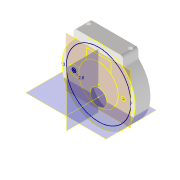
# Autodesk Inventor part: Pump_Base_Motor_tubeholder_new
Saved by Autodesk Inventor 2022.5 (Build 265521000, 521)
## iProperties
Created: 2023-11-14
Part Number: Pump_Base_Motor_tubeholder_new
Material: Generisch
Document SubType Name: Modeling
Designer: diederichbenedict
Density: 1 g/cm^3
Appearance: Vorgabe
Author: diederichbenedict
Autodesk Inventor part; units mm, degrees
ref_plane "YZ Plane" through (0, 0, 0) normal (1, 0, 0) x (0, 1, 0)
ref_plane "XZ Plane" through (0, 0, 0) normal (0, 1, 0) x (-1, 0, 0)
ref_plane "XY Plane" through (0, 0, 0) normal (0, 0, 1) x (1, 0, 0)
ref_plane "Arbeitsebene1" through (0, 0, 0) normal (0, 0, 1) x (1, 0, 0)
sketch "Skizze1" plane through (0, 0, 0) normal (0, 0, 1) x (1, 0, 0)
  arc A0 (-13.5554, 10.695) -> (13.5554, 10.695) centre (0, 14.195) ccw projected
  arc A1 (19.6, 14.195) -> (15.4, 14.195) centre (17.5, 14.195) ccw projected
  circle A2 centre (-17.5, 14.195) radius 2.1 projected
  arc A3 (4.55, 6.195) -> (-4.55, 6.195) centre (0, 6.195) ccw projected
  circle A4 centre (0, 14.195) radius 26
  circle A5 centre (-17.5, 14.195) radius 1.4
  circle A6 centre (17.5, 14.195) radius 1.4
  circle A7 centre (0, 6.195) radius 6
  point P0 (0, 0)
  dimension "d0" = 52
  dimension "d1" = 2.8
  dimension "d2" = 2.8
  dimension "d3" = 12
  constraints: 4 centre point, 4 coincident
  measures "d0" diameter of A4
  measures "d1" diameter of A5
  measures "d2" diameter of A6
  measures "d3" diameter of A7
extrude "Extrusion1" add sketch "Skizze1" against normal blind 1 contours A2 | A4
sketch "Skizze2" plane through (0, 14.195, 0) normal (0, 0, 1) x (1, 0, 0)
  circle A0 centre (0, 0) radius 26 projected
  circle A1 centre (0, -8) radius 6 projected
  circle A2 centre (17.5, 0) radius 1.4 projected
  arc A3 (14, 0) -> (-14, 0) centre (0, 0) ccw projected
  circle A4 centre (0, 0) radius 14 projected
  line L0 (-13.5554, -3.5) -> (-17.5, -3.5) projected
  arc A5 (-17.5, 3.5) -> (-17.5, -3.5) centre (-17.5, 0) ccw projected
  line L1 (-17.5, 3.5) -> (-13.5554, 3.5) projected
  line L2 (-8.75, 18.5) -> (-8.75, 10.9287) projected
  line L3 (8.75, 18.5) -> (-8.75, 18.5) projected
  line L4 (8.75, 18.5) -> (8.75, 10.9287) projected
  circle A6 centre (0, 0) radius 23
  circle A7 centre (-17.5, 0) radius 1.4
  point P0 (0, -14.195)
  dimension "d6" = 3
  dimension "d9" = 2.8
  constraints: 2 centre point, 1 coincident
  measures "d6" radial gap between concentric circles of A0 A6
  measures "d9" diameter of A7
ref_plane "Arbeitsebene2" through (-14.0001, 0.1949, 19.5) normal (0, 0, 1) x (1, 0, 0)
sketch "Skizze3" plane through (0, 14.195, -1) normal (0, 0, -1) x (-1, 0, 0)
  circle A0 centre (0, -8) radius 6 projected
  circle A1 centre (0, 0) radius 26 projected
  circle A2 centre (0, -8) radius 18
  circle A3 centre (17.5, 0) radius 1.4 projected
  circle A4 centre (-17.5, 0) radius 1.4 projected
  line L0 (17.9315, -6.4312) -> (18.9283, -17.8247)
  line L1 (-17.9315, -6.4312) -> (-18.9283, -17.8247)
  line L2 (0, 0.42) -> (0, -2.52)
  line L3 (0, 0.42) -> (0, -2.52)
  line L4 (0, 0.42) -> (0, -43.0807)
  point P0 (0, -14.195)
  point P1 (-16.6205, -1.0893)
  point P2 (-16.1008, 0.0476)
  point P3 (16.1008, 0.0476)
  point P4 (16.6205, -1.0893)
  point P5 (0, -26)
  dimension "d10" = 36
  dimension "d11" = 5
  dimension "d12" = 5
  constraints: 10 end point, 4 point on circle, 3 vertical, 2 tangent, 1 centre point, 1 coincident, 4 other
  measures "d10" diameter of A2
  measures "d11" angle of L4 L0
  measures "d12" angle of L1 L4
extrude "Extrusion3" add sketch "Skizze3" along normal blind 10 contours A1 L0 A2 A3 A4 L1 | L1 A2 A1 | A1 A2 L0
ref_plane "Arbeitsebene4" through (0, 6.195, -1) normal (0, -1, 0) x (0, 0, 1)
ref_plane "Arbeitsebene3" through (0, 25.1237, 0) normal (-1, 0, 0) x (0, 0, 1)
sketch "Skizze4" plane through (0, 6.195, -1) normal (0, -1, 0) x (0, 0, 1)
  line L0 (0, -17.9315) -> (-10, -17.9315) projected
  line L1 (-10, -18.9283) -> (-10, -16.1283)
  line L2 (-10, 26) -> (-10, -26) projected
  line L3 (-10, -16.1283) -> (-8, -16.1283)
  arc A0 (-8, -16.1283) -> (-3, -16.1283) centre (-5.5, -11.0932) ccw
  line L4 (-3, -16.1283) -> (0, -16.1283)
  line L5 (0, -16.1283) -> (0, -19.0869)
  line L6 (0, -19.0869) -> (-10, -19.0869)
  line L7 (0, 18.9283) -> (0, -18.9283) projected
  line L8 (-12.2, 0) -> (3.2, 0) projected
  line L9 (0, 16.1008) -> (0, -16.1008) construction
  line L10 (0, 16.1008) -> (-10, 16.1008) construction
  line L11 (-10, -16.1008) -> (-10, 16.1008) construction
  line L12 (0, -16.1008) -> (-10, -16.1008) construction
  point P0 (1, 0)
  point P1 (-10, 18.9283)
  point P2 (-1.5, -16.1283)
  dimension "d16" = 2.8
  dimension "d17" = 0
  dimension "d28" = 2
  dimension "d29" = 3
  constraints: 10 end point, 3 perpendicular, 3 point on line, 2 point on circle, 1 centre point, 1 horizontal, 1 midpoint
  measures "d16" distance of L1.start L1.end
  measures "d17" distance from line of point (-1.5, -16.128) L3
  measures "d28" distance from line of L2 L3.end
  measures "d29" distance from line of L7 L4.start
revolve "Umdrehung1" add sketch "Skizze4" angle 360 about axis through (0, 6.195, -1) along (0, 0, 1) contours L5 L6 L2 L1 L0 | L0 L1 L3 A0 L4 L5
sketch "Skizze7" plane through (0, 6.195, -1) normal (0, -1, 0) x (0, 0, 1)
  arc A0 (-8, -16.1283) -> (-3, -16.1283) centre (-6.5, -11.6932) ccw projected
  line L0 (-3, -16.1283) -> (-3, 16.1283) projected
  line L1 (-8, -16.1283) -> (-8, 16.1283) projected
  circle A1 centre (-6.5, -15.3148) radius 2
  circle A2 centre (-6.5, 15.3148) radius 2
  point P0 (1, 0)
  dimension "d30" = 4
  dimension "d31" = 4
  constraints: 2 centre point, 2 other
  measures "d30" diameter of A1
  measures "d31" diameter of A2
extrude "Extrusion5" cut sketch "Skizze7" along normal through all
sketch "Skizze8" plane through (0, 14.195, -11) normal (0, 0, -1) x (-1, 0, 0)
  arc A0 (-11.1651, -23.4806) -> (11.1651, -23.4806) centre (0, -8) ccw projected
  arc A1 (11.1651, -23.4806) -> (-11.1651, -23.4806) centre (0, 0) ccw projected
  arc A2 (-16.7375, 1.1742) -> (-17.8891, -1.3448) centre (-17.5, 0) ccw projected
  arc A3 (-16.7375, 1.1742) -> (-17.8891, -1.3448) centre (0, -8) ccw projected
  circle A4 centre (0, -8) radius 16.1283 projected
  arc A5 (17.8891, -1.3448) -> (16.7375, 1.1742) centre (0, -8) ccw projected
  arc A6 (17.8891, -1.3448) -> (16.7375, 1.1742) centre (17.5, 0) ccw projected
  circle A7 centre (17.5, 0) radius 1.4 projected
  point P0 (0, -14.195)
  constraints: 2 coincident
hole "Bohrung1" at (17.5, 14.195, -11) at (-17.5, 14.195, -11) at (17.5, 14.195, -11) at (-17.5, 14.195, -11) direction (0, 0, 1) diameter 3 end through all
sketch "Skizze9" plane through (0, 14.195, -11) normal (0, 0, -1) x (-1, 0, 0)
  arc A0 (-15.5, 26) -> (-17.5, 24) centre (-15.5, 24) ccw
  line L0 (-17.5, 24) -> (-17.5, 20.0935)
  arc A1 (-18.1071, 18.6583) -> (-17.5, 20.0935) centre (-19.5, 20.0935) ccw
  arc A2 (-18.1071, 18.6583) -> (18.1071, 18.6583) centre (0, 0) ccw
  arc A3 (17.5, 20.0935) -> (18.1071, 18.6583) centre (19.5, 20.0935) ccw
  line L1 (17.5, 20.0935) -> (17.5, 24)
  arc A4 (17.5, 24) -> (15.5, 26) centre (15.5, 24) ccw
  line L2 (15.5, 26) -> (-15.5, 26)
  circle A5 centre (0, -8) radius 6
  circle A6 centre (-17.5, 0) radius 1.4
  circle A7 centre (17.5, 0) radius 1.4
  circle A8 centre (17.3704, 5.3872) radius 1.4
  circle A9 centre (-5.3876, 17.37) radius 1.4
  circle A10 centre (4.938, 17.3387) radius 1.4
  circle A11 centre (-17.3391, 4.9376) radius 1.4
  arc A12 (-5.4542, -26.319) -> (-7.7325, -25.7419) centre (-5.8493, -23.0931) ccw
  arc A13 (-5.4542, -26.319) -> (18.6389, 19.3647) centre (0, -0.0004) ccw
  arc A14 (17.9875, 19.9712) -> (18.6389, 19.3647) centre (16.1194, 17.3118) ccw
  arc A15 (17.9875, 19.9712) -> (-25.8902, -7.2196) centre (0, -0.0004) ccw
  arc A16 (-25.1605, -9.4537) -> (-25.8902, -7.2196) centre (-22.645, -7.3959) ccw
  arc A17 (-25.1605, -9.4537) -> (-7.7325, -25.7419) centre (0, -0.0004) ccw
  spline S0 degree 3 poles (11.4969, 6.4027) (11.3111, 6.5852) (11.1626, 6.8022) (10.9573, 7.2809) (10.9024, 7.538) (10.8943, 8.0586) (10.9411, 8.3172) (11.1279, 8.7937) (11.2631, 9.0084) (11.4344, 9.1924) knots 0 0 0 0 0.252225 0.252225 0.504373 0.504373 0.756494 0.756494 1 1 1 1
  line L3 (11.4969, 6.4027) -> (16.3352, 1.6525)
  arc A18 (16.3628, -1.3486) -> (16.3352, 1.6525) centre (14.8485, 0.1382) ccw
  line L4 (16.3628, -1.3486) -> (1.6506, -16.3336)
  arc A19 (-1.3505, -16.3612) -> (1.6506, -16.3336) centre (0.1362, -14.8469) ccw
  line L5 (-1.3505, -16.3612) -> (-16.3355, -1.649)
  arc A20 (-16.3631, 1.3521) -> (-16.3355, -1.649) centre (-14.8488, -0.1346) ccw
  line L6 (-16.3631, 1.3521) -> (-1.6509, 16.3371)
  arc A21 (1.3502, 16.3647) -> (-1.6509, 16.3371) centre (-0.1366, 14.8504) ccw
  line L7 (1.3502, 16.3647) -> (4.6747, 13.1007)
  spline S1 degree 3 poles (7.4651, 13.0895) (7.2778, 12.9085) (7.0569, 12.7659) (6.573, 12.5733) (6.3145, 12.5252) (5.7938, 12.5308) (5.5365, 12.5845) (5.0651, 12.7838) (4.8541, 12.9246) (4.6747, 13.1007) knots 0 0 0 0 0.252231 0.252231 0.504388 0.504388 0.756517 0.756517 1 1 1 1
  arc A22 (11.4344, 9.1924) -> (7.4651, 13.0895) centre (9.3983, 11.0886) ccw
  arc A23 (24.4206, 8.9238) -> (24.4206, -8.9238) centre (0, 0) ccw
  circle A24 centre (15.0206, 14.9815) radius 1.4
  circle A25 centre (-14.9794, -15.0186) radius 1.4
  circle A26 centre (15.0206, -15.0185) radius 1.4
  circle A27 centre (-14.9794, 14.9814) radius 1.4
  point P0 (0, -14.195)
  point P1 (0, 26)
extrude "Extrusion6" add sketch "Skizze9" against normal up to surface (11 mm away) contours L2 A15 L0 A0 | L2 A23 A1 L0 A15 | L2 A15 L1 A14 A23 | L2 A4 L1 A15 | A14 L1 A3 A23
sketch "Skizze10" plane through (-15.5, 40.195, -11) normal (0, 1, 0) x (1, 0, 0)
  arc A0 (0, -29.8077) -> (0, -27.1923) centre (0.5, -28.5) ccw projected
  arc A1 (31, -27.1923) -> (31, -29.8077) centre (30.5, -28.5) ccw projected
  line L0 (0.5, -28.5) -> (30.5, -28.5)
  line L1 (30.5, -28.5) -> (30.5, -3.5)
  line L2 (30.5, -3.5) -> (0.5, -3.5)
  line L3 (0.5, -3.5) -> (0.5, -28.5)
  point P0 (15.5, -11)
  dimension "d43" = 25
  constraints: 8 end point, 2 coincident, 2 parallel, 1 horizontal, 1 perpendicular
  measures "d43" distance of L1.end L0.end
hole "Bohrung2" at (-15, 40.195, -7.5) at (15, 40.195, -7.5) direction (0, -1, 0) diameter 2.8 depth 8 tip angle 118
